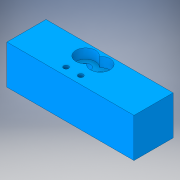
# Autodesk Inventor part: GripperBlock
Saved by Autodesk Inventor 2019 (Build 230136000, 136)
## iProperties
Created: 2019-10-02
Part Number: GripperBlock
Material: Generic
Document SubType Name: Modeling
Designer: james
Density: 1 g/cm^3
Appearance: Default(2)
Author: james
Autodesk Inventor part; units mm, degrees
ref_plane "YZ Plane" through (0, 0, 0) normal (1, 0, 0) x (0, 1, 0)
ref_plane "XZ Plane" through (0, 0, 0) normal (0, 1, 0) x (-1, 0, 0)
ref_plane "XY Plane" through (0, 0, 0) normal (0, 0, 1) x (1, 0, 0)
sketch "Sketch1" plane through (0, 0, 0) normal (1, 0, 0) x (0, 1, 0)
  line L0 (11.2985, 26.2091) -> (-39.5015, 26.2091)
  line L1 (-39.5015, 26.2091) -> (-39.5015, -24.5909)
  line L2 (-39.5015, -24.5909) -> (11.2985, -24.5909)
  line L3 (11.2985, -24.5909) -> (11.2985, 26.2091)
  point P0 (0, 0)
  dimension "d0" = 50.8
  dimension "d1" = 50.8
  constraints: 8 end point, 2 parallel, 1 horizontal, 1 perpendicular
  measures "d0" distance of L2.end L0.start
  measures "d1" distance of L0.start L0.end
extrude "Extrusion1" add sketch "Sketch1" along normal blind 165.1
sketch "Sketch2" plane through (0, 11.2985, 26.2091) normal (0, 1, 0) x (1, 0, 0)
  circle A0 centre (66.675, 35.56) radius 12.7
  circle A1 centre (85.725, 35.56) radius 12.7
  line L0 (0, 50.8) -> (0, 0) projected
  line L1 (0, 50.8) -> (165.1, 50.8) projected
  point P0 (0, 26.2091)
  dimension "d4" = 25.4
  dimension "d5" = 25.4
  dimension "d6" = 0
  dimension "d7" = 19.05
  dimension "d8" = 66.675
  dimension "d9" = 15.24
  constraints: 2 centre point
  measures "d4" diameter of A0
  measures "d5" diameter of A1
  measures "d6" vertical distance of A0.centre A1.centre
  measures "d7" distance of A0.centre A1.centre
  measures "d8" distance from line of L0 A0.centre
  measures "d9" distance from line of L1 A0.centre
extrude "Extrusion2" cut sketch "Sketch2" against normal blind 12.7
sketch "Sketch3" plane through (0, -1.4015, 26.2091) normal (0, 1, 0) x (1, 0, 0)
  arc A0 (76.2, 27.1597) -> (76.2, 43.9603) centre (85.725, 35.56) ccw projected
  arc A1 (76.2, 43.9603) -> (76.2, 27.1597) centre (66.675, 35.56) ccw projected
  circle A2 centre (66.675, 35.56) radius 3.302
  circle A3 centre (85.725, 35.56) radius 3.302
  point P0 (0, 26.2091)
  dimension "d12" = 6.604
  dimension "d13" = 6.604
  constraints: 2 centre point, 2 coincident
  measures "d12" diameter of A2
  measures "d13" diameter of A3
extrude "Extrusion3" cut sketch "Sketch3" against normal blind 76.2 contours A2 | A3
sketch "Sketch4" plane through (0, -39.5015, -24.5909) normal (0, -1, 0) x (1, 0, 0)
  circle A0 centre (66.675, 15.24) radius 3.302 projected
  circle A1 centre (85.725, 15.24) radius 3.302 projected
  line L0 (0, 50.8) -> (0, 0) projected
  line L1 (0, 0) -> (165.1, 0) projected
  line L2 (165.1, 50.8) -> (165.1, 0) projected
  line L3 (0, 50.8) -> (165.1, 50.8) projected
  circle A2 centre (85.725, 15.24) radius 3.302 projected
  circle A3 centre (66.675, 15.24) radius 12.7
  circle A4 centre (85.725, 15.24) radius 12.7
  point P0 (0, 24.5909)
  dimension "d16" = 25.4
  dimension "d17" = 25.4
  constraints: 2 centre point, 2 coincident
  measures "d16" diameter of A4
  measures "d17" diameter of A3
extrude "Extrusion4" cut sketch "Sketch4" against normal blind 12.7 contours A3 A4 | A3 A4 | A4 A3
sketch "Sketch5" plane through (0, -26.8015, -24.5909) normal (0, -1, 0) x (1, 0, 0)
  circle A0 centre (66.675, 15.24) radius 3.302 projected
  circle A1 centre (85.725, 15.24) radius 3.302 projected
  circle A2 centre (66.675, 15.24) radius 6.35
  circle A3 centre (85.725, 15.24) radius 6.35
  point P0 (0, 24.5909)
  dimension "d20" = 12.7
  dimension "d21" = 12.7
  constraints: 2 centre point, 2 coincident
  measures "d20" diameter of A2
  measures "d21" diameter of A3
extrude "Extrusion5" cut sketch "Sketch5" against normal blind 6.35
sketch "Sketch6" plane through (0, -1.4015, 26.2091) normal (0, 1, 0) x (1, 0, 0)
  circle A0 centre (66.675, 35.56) radius 3.302 projected
  circle A1 centre (85.725, 35.56) radius 3.302 projected
  circle A2 centre (66.675, 35.56) radius 6.35
  circle A3 centre (85.725, 35.56) radius 6.35
  point P0 (0, 26.2091)
  dimension "d24" = 12.7
  dimension "d25" = 12.7
  constraints: 2 centre point, 2 coincident
  measures "d24" diameter of A2
  measures "d25" diameter of A3
extrude "Extrusion6" cut sketch "Sketch6" against normal blind 6.35
sketch "Sketch7" plane through (0, -39.5015, -24.5909) normal (0, -1, 0) x (1, 0, 0)
  circle A0 centre (66.675, 40.64) radius 3.175
  circle A1 centre (85.725, 40.64) radius 3.175
  circle A2 centre (66.675, 15.24) radius 3.302 projected
  circle A3 centre (85.725, 15.24) radius 3.302 projected
  point P0 (0, 24.5909)
  dimension "d28" = 6.35
  dimension "d29" = 6.35
  dimension "d30" = 19.05
  dimension "d31" = 0
  dimension "d32" = 25.4
  dimension "d33" = 25.4
  constraints: 2 centre point
  measures "d28" diameter of A0
  measures "d29" diameter of A1
  measures "d30" distance of A0.centre A1.centre
  measures "d31" horizontal distance of A2.centre A0.centre
  measures "d32" distance of A0.centre A2.centre
  measures "d33" distance of A3.centre A1.centre
extrude "Extrusion7" cut sketch "Sketch7" against normal blind 76.2 contours A0 | A1
body "Solid1"
